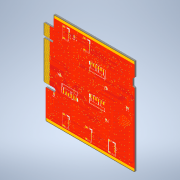
# Autodesk Inventor part: Avionics_PCB
Saved by Autodesk Inventor 2021 (Build 250183000, 183)
## iProperties
Created: 2018-01-15
Part Number: Avionics_PCB
Material: Epoxy Resin
Document SubType Name: Modeling
Designer: Bradley
Density: 1.14 g/cm^3
Appearance: Smooth - Medium Gray
Mass: 15.4834 g
Surface Area: 175.95 cm^2
Volume: 13.582 cm^3
Author: Bradley
Revision Number: 3.1
Autodesk Inventor part; units mm, degrees
ref_plane "XZ Plane" through (0, 0, 0) normal (0, 1, 0) x (-1, 0, 0)
ref_plane "XY Plane" through (0, 0, 0) normal (0, 0, 1) x (1, 0, 0)
sketch "Sketch1" plane through (0, 0, 0) normal (0, 0, 1) x (1, 0, 0)
  line L0 (0, 36.15) -> (10, 36.15)
  line L1 (10, 36.15) -> (10, 47.9)
  line L2 (10, 47.9) -> (90.4, 47.9)
  line L3 (90.4, 47.9) -> (90.4, -47.9)
  line L4 (90.4, -47.9) -> (2, -47.9)
  line L5 (10, -15.15) -> (0, -15.15)
  line L6 (-5.5, 48) -> (90.5, 48) construction
  line L7 (90.5, 48) -> (90.5, -48) construction
  line L8 (90.5, -48) -> (-5.5, -48) construction
  line L9 (-5.5, -48) -> (-5.5, 48) construction
  line L10 (-5.4, 47.9) -> (-3.4, 47.9) construction
  line L11 (-3.4, 47.9) -> (-3.4, -47.9) construction
  line L12 (-3.4, -47.9) -> (-5.4, -47.9) construction
  line L13 (-5.4, -47.9) -> (-5.4, 47.9) construction
  line L14 (-3.4, 38.5) -> (7.85, 38.5) construction
  line L15 (7.85, 38.5) -> (7.85, -17.5) construction
  line L16 (7.85, -17.5) -> (-3.4, -17.5) construction
  line L17 (-3.4, -17.5) -> (-3.4, 38.5) construction
  line L18 (2, -47.9) -> (2, -18.65)
  line L19 (2, -18.65) -> (10, -18.65)
  arc A0 (10, -18.65) -> (10, -15.15) centre (10, -16.9) ccw
  line L20 (0, 24) -> (90.5, 24) construction
  circle A1 centre (-2.5, 47.1) radius 0.9 construction
  circle A2 centre (-0.7, 47.1) radius 0.9 construction
  circle A3 centre (1.1, 47.1) radius 0.9 construction
  circle A4 centre (2.9, 47.1) radius 0.9 construction
  circle A5 centre (4.7, 47.1) radius 0.9 construction
  circle A6 centre (6.5, 47.1) radius 0.9 construction
  circle A7 centre (8.3, 47.1) radius 0.9 construction
  circle A8 centre (-2.5, 45.3) radius 0.9 construction
  circle A9 centre (-0.7, 45.3) radius 0.9 construction
  circle A10 centre (1.1, 45.3) radius 0.9 construction
  circle A11 centre (2.9, 45.3) radius 0.9 construction
  circle A12 centre (4.7, 45.3) radius 0.9 construction
  circle A13 centre (6.5, 45.3) radius 0.9 construction
  circle A14 centre (8.3, 45.3) radius 0.9 construction
  circle A15 centre (-2.5, 43.5) radius 0.9 construction
  circle A16 centre (-0.7, 43.5) radius 0.9 construction
  circle A17 centre (1.1, 43.5) radius 0.9 construction
  circle A18 centre (2.9, 43.5) radius 0.9 construction
  circle A19 centre (4.7, 43.5) radius 0.9 construction
  circle A20 centre (6.5, 43.5) radius 0.9 construction
  circle A21 centre (8.3, 43.5) radius 0.9 construction
  circle A22 centre (-2.5, 41.7) radius 0.9 construction
  circle A23 centre (-0.7, 41.7) radius 0.9 construction
  circle A24 centre (1.1, 41.7) radius 0.9 construction
  circle A25 centre (2.9, 41.7) radius 0.9 construction
  circle A26 centre (4.7, 41.7) radius 0.9 construction
  circle A27 centre (6.5, 41.7) radius 0.9 construction
  circle A28 centre (8.3, 41.7) radius 0.9 construction
  circle A29 centre (-2.5, 39.9) radius 0.9 construction
  circle A30 centre (-0.7, 39.9) radius 0.9 construction
  circle A31 centre (1.1, 39.9) radius 0.9 construction
  circle A32 centre (2.9, 39.9) radius 0.9 construction
  circle A33 centre (4.7, 39.9) radius 0.9 construction
  circle A34 centre (6.5, 39.9) radius 0.9 construction
  circle A35 centre (8.3, 39.9) radius 0.9 construction
  line L21 (0, 36.15) -> (0, 24.95)
  line L22 (0, 24.95) -> (8.4, 24.95)
  arc A36 (8.4, 23.05) -> (8.4, 24.95) centre (8.4, 24) ccw
  line L23 (8.4, 23.05) -> (0, 23.05)
  line L24 (0, 23.05) -> (0, -15.15)
  point P0 (0, 0)
  point P1 (-5.5, 0)
  point P2 (90.4, 0)
  point P3 (90.5, 0)
  dimension "d0" = 51.3
  dimension "d1" = 95.8
  dimension "d3" = 10
  dimension "d20" = 96
  dimension "d21" = 96
  dimension "d22" = 0.1
  dimension "d23" = 0.1
  dimension "d24" = 2
  dimension "d25" = 0.1
  dimension "d28" = 11.25
  dimension "d29" = 56
  dimension "d31" = 9.5
  dimension "d32" = 30.5
  dimension "d34" = 3.5
  dimension "d35" = 12.15
  dimension "d36" = 39.15
  dimension "d37" = 14.5
  dimension "d38" = 1.15
  dimension "d39" = 1.8
  dimension "d42" = 1.8
  dimension "d45" = 1.8
  dimension "d48" = 2
  dimension "d49" = 3.4
  dimension "d50" = 1.9
  dimension "d51" = 8.4
  dimension "d52" = 24
  constraints: 50 end point, 37 centre point, 11 perpendicular, 7 parallel, 6 point on line, 6 tangent, 5 horizontal, 4 point on circle, 3 midpoint, 3 vertical, 2 collinear, 2 horizontal alignment, 68 other
  measures "d0" distance of L5.end L0.start
  measures "d1" distance of L2.end L3.end
  measures "d3" distance of L0.start L0.end
  measures "d20" distance of L6.start L6.end
  measures "d21" distance of L8.end L6.start
  measures "d22" distance between parallel lines of L2 L6
  measures "d23" distance between parallel lines of L7 L3
  measures "d24" distance between parallel lines of L13 L11
  measures "d25" distance between parallel lines of L13 L9
  measures "d28" distance of L15.end L16.end
  measures "d29" distance of L14.end L15.end
  measures "d31" distance between parallel lines of L14 L6
  measures "d32" distance between parallel lines of L8 L16
  measures "d34" distance between parallel lines of L5 L19
  measures "d35" distance between parallel lines of L20 L0
  measures "d36" distance between parallel lines of L5 L20
  measures "d37" distance between parallel lines of L20 L14
  measures "d38" distance between parallel lines of L19 L16
  measures "d39" diameter of A1
  measures "d42" distance of A1.centre A2.centre
  measures "d45" distance of A1.centre A8.centre
  measures "d48" distance between parallel lines of L18 L24
  measures "d49" distance between parallel lines of L24 L11
  measures "d50" distance between parallel lines of L23 L22
  measures "d51" distance of L21.end L22.end
  measures "d52" distance from line of point (0, 0) L20
extrude "Extrusion1" add sketch "Sketch1" along normal mid plane 1.6
chamfer "Chamfer1" distance 0.5 angle 45 4 edges at (0, 36.15, 0) (0, 24.95, 0) (0, 23.05, 0) (0, -15.15, 0)
fillet "Fillet1" radius 0.5 6 edges at (10, 36.15, 0) (10, 47.9, 0) (90.4, 47.9, 0) (90.4, -47.9, 0) (2, -47.9, 0) (2, -18.65, 0)
sketch "Sketch16" plane through (0, 0, 0.8) normal (0, 0, 1) x (1, 0, 0)
  arc A0 (2.5, -18.65) -> (2, -19.15) centre (2.5, -19.15) ccw projected
  line L0 (2, -19.15) -> (2, -47.4) projected
  arc A1 (2, -47.4) -> (2.5, -47.9) centre (2.5, -47.4) ccw projected
  line L1 (2.5, -47.9) -> (89.9, -47.9) projected
  arc A2 (89.9, -47.9) -> (90.4, -47.4) centre (89.9, -47.4) ccw projected
  line L2 (90.4, -47.4) -> (90.4, 47.4) projected
  arc A3 (90.4, 47.4) -> (89.9, 47.9) centre (89.9, 47.4) ccw projected
  line L3 (89.9, 47.9) -> (10.5, 47.9) projected
  arc A4 (10.5, 47.9) -> (10, 47.4) centre (10.5, 47.4) ccw projected
  line L4 (10, 47.4) -> (10, 36.65) projected
  arc A5 (9.5, 36.15) -> (10, 36.65) centre (9.5, 36.65) ccw projected
  line L5 (9.5, 36.15) -> (0.5, 36.15) projected
  line L6 (0, 35.65) -> (0.5, 36.15) projected
  line L7 (0, 35.65) -> (0, 25.45) projected
  line L8 (0.5, 24.95) -> (0, 25.45) projected
  line L9 (0.5, 24.95) -> (8.4, 24.95) projected
  arc A6 (8.4, 23.05) -> (8.4, 24.95) centre (8.4, 24) ccw projected
  line L10 (8.4, 23.05) -> (0.5, 23.05) projected
  line L11 (0, 22.55) -> (0.5, 23.05) projected
  line L12 (0, 22.55) -> (0, -14.65) projected
  line L13 (0.5, -15.15) -> (0, -14.65) projected
  line L14 (0.5, -15.15) -> (10, -15.15) projected
  arc A7 (10, -18.65) -> (10, -15.15) centre (10, -16.9) ccw projected
  line L15 (10, -18.65) -> (2.5, -18.65) projected
  line L16 (90.4, -47.4) -> (90.4, 47.4) projected
  arc A8 (89.4, 33) -> (90.4, 34) centre (89.4, 34) ccw
  arc A9 (89.4, 33) -> (88.4, 32) centre (89.4, 32) ccw
  arc A10 (88.4, 26) -> (89.4, 25) centre (89.4, 26) ccw
  arc A11 (90.4, 24) -> (89.4, 25) centre (89.4, 24) ccw
  line L17 (88.4, 32) -> (88.4, 26)
  line L18 (88.4, 29) -> (90.4, 29) construction
  point P0 (0, 0)
  dimension "d145" = 1
  dimension "d146" = 29
  dimension "d147" = 8
  dimension "d148" = 34
  constraints: 8 point on circle, 6 tangent, 4 centre point, 4 end point, 3 equal radius, 3 point on line, 1 midpoint, 1 perpendicular, 1 vertical, 1 vertical alignment
  measures "d145" radius of A11
  measures "d146" distance from line of L18 point (0, 0)
  measures "d147" distance of A10.end A8.start
  measures "d148" vertical distance of point (0, 0) A8.end
extrude "Extrusion6" cut sketch "Sketch16" against normal through all contours A11 A10 L17 A9 A8 L2
ref_plane "Work Plane1" through (4, 0, 0) normal (1, 0, 0) x (0, 1, 0)
sketch "Sketch17" plane through (4, 0, 0) normal (1, 0, 0) x (0, 1, 0)
  line L0 (-19.15, -0.8) -> (-19.15, 0.8) projected
  line L1 (-47.4, -0.8) -> (-19.15, -0.8) projected
  line L2 (-47.4, 0.8) -> (-47.4, -0.8) projected
  line L3 (-19.15, 0.8) -> (-47.4, 0.8) projected
  point P0 (0, 0)
  point P1 (-42, 1.8)
  point P2 (-41, 1.8)
  point P3 (-40, 1.8)
  point P4 (-39, 1.8)
  point P5 (-42, 2.8)
  point P6 (-41, 2.8)
  point P7 (-40, 2.8)
  point P8 (-39, 2.8)
  point P9 (-42, 3.8)
  point P10 (-41, 3.8)
  point P11 (-40, 3.8)
  point P12 (-39, 3.8)
  point P13 (-42, 4.8)
  point P14 (-41, 4.8)
  point P15 (-40, 4.8)
  point P16 (-39, 4.8)
  dimension "d154" = 1
  dimension "d157" = 1
  dimension "d160" = 42
  dimension "d161" = 1
  constraints: 1 horizontal, 1 vertical, 15 other
  measures "d154" distance of point (-42, 1.8) point (-41, 1.8)
  measures "d157" distance of point (-42, 1.8) point (-42, 2.8)
  measures "d160" horizontal distance of point (-42, 1.8) point (0, 0)
  measures "d161" distance from line of L3 point (-42, 1.8)
sketch "Sketch18" plane through (0, 0, 0) normal (0, 0, 1) x (1, 0, 0)
  arc A0 (90.4, 24) -> (89.4, 25) centre (89.4, 24) ccw projected
  arc A1 (88.4, 26) -> (89.4, 25) centre (89.4, 26) ccw projected
  line L0 (88.4, 26) -> (88.4, 32) projected
  arc A2 (89.4, 33) -> (88.4, 32) centre (89.4, 32) ccw projected
  arc A3 (89.4, 33) -> (90.4, 34) centre (89.4, 34) ccw projected
  line L1 (90.4, 34) -> (90.4, 47.4) projected
  arc A4 (90.4, 47.4) -> (89.9, 47.9) centre (89.9, 47.4) ccw projected
  line L2 (89.9, 47.9) -> (10.5, 47.9) projected
  arc A5 (10.5, 47.9) -> (10, 47.4) centre (10.5, 47.4) ccw projected
  line L3 (10, 47.4) -> (10, 36.65) projected
  arc A6 (9.5, 36.15) -> (10, 36.65) centre (9.5, 36.65) ccw projected
  line L4 (9.5, 36.15) -> (0.5, 36.15) projected
  line L5 (0, 35.65) -> (0.5, 36.15) projected
  line L6 (0, 35.65) -> (0, 25.45) projected
  line L7 (0.5, 24.95) -> (0, 25.45) projected
  line L8 (0.5, 24.95) -> (8.4, 24.95) projected
  arc A7 (8.4, 23.05) -> (8.4, 24.95) centre (8.4, 24) ccw projected
  line L9 (8.4, 23.05) -> (0.5, 23.05) projected
  line L10 (0, 22.55) -> (0.5, 23.05) projected
  line L11 (0, 22.55) -> (0, -14.65) projected
  line L12 (0.5, -15.15) -> (0, -14.65) projected
  line L13 (0.5, -15.15) -> (10, -15.15) projected
  arc A8 (10, -18.65) -> (10, -15.15) centre (10, -16.9) ccw projected
  line L14 (10, -18.65) -> (2.5, -18.65) projected
  arc A9 (2.5, -18.65) -> (2, -19.15) centre (2.5, -19.15) ccw projected
  line L15 (2, -19.15) -> (2, -47.4) projected
  arc A10 (2, -47.4) -> (2.5, -47.9) centre (2.5, -47.4) ccw projected
  line L16 (2.5, -47.9) -> (89.9, -47.9) projected
  arc A11 (89.9, -47.9) -> (90.4, -47.4) centre (89.9, -47.4) ccw projected
  line L17 (90.4, -47.4) -> (90.4, 24) projected
  point P0 (0, 0)
  point P1 (1.5, -44.9)
  point P2 (0.5, -44.9)
  point P3 (1.5, -43.9)
  point P4 (0.5, -43.9)
  point P5 (1.5, -42.9)
  point P6 (0.5, -42.9)
  point P7 (1.5, -41.9)
  point P8 (0.5, -41.9)
  point P9 (1.5, -40.9)
  point P10 (0.5, -40.9)
  point P11 (1.5, -39.9)
  point P12 (0.5, -39.9)
  point P13 (1.5, -38.9)
  point P14 (0.5, -38.9)
  point P15 (1.5, -37.9)
  point P16 (0.5, -37.9)
  point P17 (1.5, -36.9)
  point P18 (0.5, -36.9)
  point P19 (1.5, -35.9)
  point P20 (0.5, -35.9)
  point P21 (1.5, -34.9)
  point P22 (0.5, -34.9)
  point P23 (1.5, -33.9)
  point P24 (0.5, -33.9)
  point P25 (1.5, -32.9)
  point P26 (0.5, -32.9)
  point P27 (1.5, -31.9)
  point P28 (0.5, -31.9)
  point P29 (1.5, -30.9)
  point P30 (0.5, -30.9)
  point P31 (1.5, -29.9)
  point P32 (0.5, -29.9)
  point P33 (1.5, -28.9)
  point P34 (0.5, -28.9)
  point P35 (1.5, -27.9)
  point P36 (0.5, -27.9)
  point P37 (1.5, -26.9)
  point P38 (0.5, -26.9)
  point P39 (1.5, -25.9)
  point P40 (0.5, -25.9)
  point P41 (1.5, -24.9)
  point P42 (0.5, -24.9)
  point P43 (1.5, -23.9)
  point P44 (0.5, -23.9)
  point P45 (1.5, -22.9)
  point P46 (0.5, -22.9)
  point P47 (1.5, -21.9)
  point P48 (0.5, -21.9)
  point P49 (1.5, -20.9)
  point P50 (0.5, -20.9)
  point P51 (9.5, 37.9)
  point P52 (9.5, 38.9)
  point P53 (9.5, 39.9)
  point P54 (9.5, 40.9)
  point P55 (9.5, 41.9)
  point P56 (9.5, 42.9)
  point P57 (9.5, 43.9)
  point P58 (8.5, 37.9)
  point P59 (8.5, 38.9)
  point P60 (8.5, 39.9)
  point P61 (8.5, 40.9)
  point P62 (8.5, 41.9)
  point P63 (8.5, 42.9)
  point P64 (8.5, 43.9)
  point P65 (7.5, 37.9)
  point P66 (7.5, 38.9)
  point P67 (7.5, 39.9)
  point P68 (7.5, 40.9)
  point P69 (7.5, 41.9)
  point P70 (7.5, 42.9)
  point P71 (7.5, 43.9)
  point P72 (6.5, 37.9)
  point P73 (6.5, 38.9)
  point P74 (6.5, 39.9)
  point P75 (6.5, 40.9)
  point P76 (6.5, 41.9)
  point P77 (6.5, 42.9)
  point P78 (6.5, 43.9)
  dimension "d164" = 1
  dimension "d167" = 1
  dimension "d170" = 0.5
  dimension "d171" = 3
  dimension "d172" = 0.5
  dimension "d173" = 10
  dimension "d176" = 1
  dimension "d179" = 1
  constraints: 2 horizontal, 2 vertical, 76 other
  measures "d164" distance of point (1.5, -44.9) point (0.5, -44.9)
  measures "d167" distance of point (1.5, -44.9) point (1.5, -43.9)
  measures "d170" distance from line of L15 point (1.5, -44.9)
  measures "d171" distance from line of L16 point (1.5, -44.9)
  measures "d172" distance from line of point (9.5, 37.9) L3
  measures "d173" distance from line of point (9.5, 37.9) L2
  measures "d176" distance of point (9.5, 37.9) point (9.5, 38.9)
  measures "d179" distance of point (9.5, 37.9) point (8.5, 37.9)
sketch "Sketch19" plane through (0, 0, 0.8) normal (0, 0, 1) x (1, 0, 0)
  line L0 (0, 22.55) -> (0, -14.65) projected
  line L1 (90.4, -47.4) -> (90.4, 24) projected
  line L2 (0, 47.8949) -> (90.4, 47.8949) construction
  line L3 (90.4, 47.8949) -> (90.4, -47.8949) construction
  line L4 (90.4, -47.8949) -> (0, -47.8949) construction
  line L5 (0, -47.8949) -> (0, 47.8949) construction
  point P0 (0, 0)
  constraints: 2 collinear, 1 midpoint, 2 other
decal "Decal3"
sketch "Sketch20" plane through (0, 0, -0.8) normal (0, 0, -1) x (-1, 0, 0)
  line L0 (0, -14.65) -> (0, 22.55) projected
  line L1 (-90.4, 24) -> (-90.4, -47.4) projected
  line L2 (-90.4, 47.8949) -> (0, 47.8949) construction
  line L3 (0, 47.8949) -> (0, -47.8949) construction
  line L4 (0, -47.8949) -> (-90.4, -47.8949) construction
  line L5 (-90.4, -47.8949) -> (-90.4, 47.8949) construction
  point P0 (0, 0)
  constraints: 2 collinear, 1 midpoint, 2 other
decal "Decal4"
sketch "Sketch22" plane through (0, 0, 0.8) normal (0, 0, 1) x (1, 0, 0)
  point P0 (0, 0)
  point P1 (6, 34.5)
  point P2 (6, 32.5)
  point P3 (6, 31.5)
  point P4 (6, 29.5)
  point P5 (6, 28.5)
  point P6 (6, 27.5)
  point P7 (6, 26.5)
  point P8 (6, 25.6)
  point P9 (6, 22.425)
  point P10 (6, 21.5)
  point P11 (6, 20.5)
  point P12 (6, 19.5)
  point P13 (6, 18.5)
  point P14 (6, 17.5)
  point P15 (6, 16.6)
  point P16 (6, 14.5)
  point P17 (6, 13.5)
  point P18 (6, 12.5)
  point P19 (6, 11.5)
  point P20 (87.9, 18.2)
  point P21 (82.2, 16.791)
  point P22 (87.6, 15.5)
  point P23 (25.3, 13.6)
  point P24 (71.8, 15.6)
  point P25 (50.2, 46.1)
  point P26 (46.2, -44.52)
  point P27 (77.9, 4.8)
  point P28 (87.2, -4.3)
  point P29 (49.9, -17.3)
  point P30 (17.6, -12.9)
  point P31 (66.5, -3)
  point P32 (65.93, -8.32)
  point P33 (48.1, 26.5)
  point P34 (66.35, 24.9)
  point P35 (26.962, -21.548)
  point P36 (32.2, -20.55)
  point P37 (65.8, 17.9)
  point P38 (66, 21.9)
  point P39 (15.4, 26.5)
  point P40 (25.9, 16.7)
  point P41 (29.235, 13.76)
  point P42 (33.1, 26.6)
  point P43 (34.7, 23.7)
  point P44 (31.5, 11.8)
  point P45 (20.9, 21.9)
  point P46 (17.7, 22.8)
  point P47 (38.325, 22.345)
  point P48 (10.995, 12.485)
  point P49 (10.995, 11.67)
  point P50 (10.3, 11.7)
  point P51 (24.31, 9)
  point P52 (23.835, 2.255)
  point P53 (33.305, -1.33)
  point P54 (35.5, -3.4)
  point P55 (29.2, -37.9)
  point P56 (46.1, -37.9)
  point P57 (63, -38.5)
  point P58 (79.9, -39.3)
  point P59 (74.3, -38.9)
  point P60 (8.61, -29.3)
  point P61 (23.5, -38.9)
  point P62 (28.3, -31)
  point P63 (39.9, -39)
  point P64 (85.5, -0.8)
  point P65 (57.89, -10.4)
  point P66 (55.74, -17.51)
  point P67 (58.4, -17.7)
  point P68 (64.9, 33.2)
  point P69 (58.25, 10.5)
  point P70 (56.85, 10.5)
  point P71 (77.1, -30.9)
  point P72 (23.425, 25.595)
  point P73 (18.9, 31.2)
  point P74 (35.465, 18.9)
  point P75 (34.135, 15.025)
  point P76 (30.15, 22.355)
  point P77 (57.35, -36.505)
  point P78 (62.1, -30.9)
  point P79 (12.855, -36.35)
  point P80 (45.2, -30.8)
  point P81 (21.925, -18.495)
  point P82 (23.935, -18.495)
  point P83 (26.315, -12.9)
  point P84 (55.3, -0.89)
  point P85 (52.8, -4.31)
  point P86 (45.6, -7.01)
  point P87 (53.275, -18.425)
  point P88 (48.555, 6.31)
  point P89 (51.785, 10.414)
  point P90 (49.681, 11.119)
  point P91 (58.92, 27.11)
  point P92 (56.4, 27.2)
  point P93 (51.67, 28.16)
  point P94 (28.745, -0.49)
  point P95 (45.439, 20.63)
  point P96 (50.617, 22.73)
  point P97 (42.571, 27.565)
  point P98 (39.712, 25.565)
  point P99 (30.035, -16.35)
  point P100 (33.621, -12.379)
  point P101 (15.835, 9)
  point P102 (18.4, -2)
  point P103 (18.4, -5)
  point P104 (24.045, -15.705)
  point P105 (48.7, 31.647)
  point P106 (52.39, 30.62)
  point P107 (70.895, 33.296)
  point P108 (81.9, 40.1)
  point P109 (37.4, 32.3)
  point P110 (24.77, 27.9)
  point P111 (80, -43)
  point P112 (63, -43)
  point P113 (40, -43)
  point P114 (8.5, -42.3)
  point P115 (15, -43)
  point P116 (18, -43)
  point P117 (85, -35)
  point P118 (85, -30)
  point P119 (85, -25)
  point P120 (85, -20)
  point P121 (85, -15)
  point P122 (85, -10)
  point P123 (80, -35)
  point P124 (80, -30)
  point P125 (80, -25)
  point P126 (80, -20)
  point P127 (80, -15)
  point P128 (73.6, -10)
  point P129 (70, -10)
  point P130 (70, -15)
  point P131 (70, -20)
  point P132 (75, -20)
  point P133 (75, -15)
  point P134 (65, -15)
  point P135 (65, -20)
  point P136 (60, -20)
  point P137 (60, -15)
  point P138 (70, -25)
  point P139 (70, -30)
  point P140 (65, -30)
  point P141 (60, -30)
  point P142 (55, -30)
  point P143 (50, -30)
  point P144 (40, -30)
  point P145 (65, -25)
  point P146 (60, -25)
  point P147 (60, -35)
  point P148 (50, -40)
  point P149 (55, -40.1)
  point P150 (35, -30)
  point P151 (35, -25)
  point P152 (25, -30)
  point P153 (30, -30)
  point P154 (30, -40)
  point P155 (21, -40)
  point P156 (20, -30)
  point P157 (15, -30)
  point P158 (15, -34)
  point P159 (5, -30)
  point P160 (5, -25)
  point P161 (5, -20)
  point P162 (15, -25)
  point P163 (20, -20)
  point P164 (25, -25)
  point P165 (30, -25)
  point P166 (30, -20)
  point P167 (35, -20)
  point P168 (45, -20)
  point P169 (40, -20)
  point P170 (40, -15)
  point P171 (45.1, -10)
  point P172 (50, -10)
  point P173 (55, -10)
  point P174 (30, 5)
  point P175 (35, 5)
  point P176 (40, 5)
  point P177 (45, 5)
  point P178 (50.2, 5)
  point P179 (55, 5)
  point P180 (60, 5)
  point P181 (65, 5)
  point P182 (65, 0)
  point P183 (50, 0)
  point P184 (70, 0)
  point P185 (70, -5)
  point P186 (65, 10)
  point P187 (85, 5)
  point P188 (85, 10)
  point P189 (65, 14)
  point P190 (40, 15)
  point P191 (44.7, 15)
  point P192 (35, 15)
  point P193 (40, 10)
  point P194 (35, 10)
  point P195 (30, 10)
  point P196 (25, 10)
  point P197 (10, 15)
  point P198 (15, 15)
  point P199 (15, 20)
  constraints: 744 other
hole "Hole10" at (6, 34.5, 0.8) at (6, 32.5, 0.8) at (6, 31.5, 0.8) at (6, 29.5, 0.8) at (6, 28.5, 0.8) at (6, 27.5, 0.8) at (6, 26.5, 0.8) at (6, 25.6, 0.8) at (6, 22.425, 0.8) at (6, 21.5, 0.8) at (6, 20.5, 0.8) at (6, 19.5, 0.8) at (6, 18.5, 0.8) at (6, 17.5, 0.8) at (6, 16.6, 0.8) at (6, 14.5, 0.8) at (6, 13.5, 0.8) at (6, 12.5, 0.8) at (6, 11.5, 0.8) at (87.9, 18.2, 0.8) at (82.2, 16.791, 0.8) at (87.6, 15.5, 0.8) at (25.3, 13.6, 0.8) at (71.8, 15.6, 0.8) at (50.2, 46.1, 0.8) at (46.2, -44.52, 0.8) at (77.9, 4.8, 0.8) at (87.2, -4.3, 0.8) at (49.9, -17.3, 0.8) at (17.6, -12.9, 0.8) at (66.5, -3, 0.8) at (65.93, -8.32, 0.8) at (48.1, 26.5, 0.8) at (66.35, 24.9, 0.8) at (26.962, -21.548, 0.8) at (32.2, -20.55, 0.8) at (65.8, 17.9, 0.8) at (66, 21.9, 0.8) at (15.4, 26.5, 0.8) at (25.9, 16.7, 0.8) at (29.235, 13.76, 0.8) at (33.1, 26.6, 0.8) at (34.7, 23.7, 0.8) at (31.5, 11.8, 0.8) at (20.9, 21.9, 0.8) at (17.7, 22.8, 0.8) at (38.325, 22.345, 0.8) at (10.995, 12.485, 0.8) at (10.995, 11.67, 0.8) at (10.3, 11.7, 0.8) direction (0, 0, -1) diameter 0.3 end through all and at (24.31, 9, 0.8) (23.835, 2.255, 0.8) (33.305, -1.33, 0.8) (35.5, -3.4, 0.8) (29.2, -37.9, 0.8) (46.1, -37.9, 0.8) (63, -38.5, 0.8) (79.9, -39.3, 0.8) (74.3, -38.9, 0.8) (8.61, -29.3, 0.8) (23.5, -38.9, 0.8) (28.3, -31, 0.8) (39.9, -39, 0.8) (85.5, -0.8, 0.8) (57.89, -10.4, 0.8) (55.74, -17.51, 0.8) (58.4, -17.7, 0.8) (64.9, 33.2, 0.8) (58.25, 10.5, 0.8) (56.85, 10.5, 0.8) (77.1, -30.9, 0.8) (23.425, 25.595, 0.8) (18.9, 31.2, 0.8) (35.465, 18.9, 0.8) (34.135, 15.025, 0.8) (30.15, 22.355, 0.8) (57.35, -36.505, 0.8) (62.1, -30.9, 0.8) (12.855, -36.35, 0.8) (45.2, -30.8, 0.8) (21.925, -18.495, 0.8) (23.935, -18.495, 0.8) (26.315, -12.9, 0.8) (55.3, -0.89, 0.8) (52.8, -4.31, 0.8) (45.6, -7.01, 0.8) (53.275, -18.425, 0.8) (48.555, 6.31, 0.8) (51.785, 10.414, 0.8) (49.681, 11.119, 0.8) (58.92, 27.11, 0.8) (56.4, 27.2, 0.8) (51.67, 28.16, 0.8) (28.745, -0.49, 0.8) (45.439, 20.63, 0.8) (50.617, 22.73, 0.8) (42.571, 27.565, 0.8) (39.712, 25.565, 0.8) (30.035, -16.35, 0.8) (33.621, -12.379, 0.8) (15.835, 9, 0.8) (18.4, -2, 0.8) (18.4, -5, 0.8) (24.045, -15.705, 0.8) (48.7, 31.647, 0.8) (52.39, 30.62, 0.8) (70.895, 33.296, 0.8) (81.9, 40.1, 0.8) (37.4, 32.3, 0.8) (24.77, 27.9, 0.8) (80, -43, 0.8) (63, -43, 0.8) (40, -43, 0.8) (8.5, -42.3, 0.8) (15, -43, 0.8) (18, -43, 0.8) (85, -35, 0.8) (85, -30, 0.8) (85, -25, 0.8) (85, -20, 0.8) (85, -15, 0.8) (85, -10, 0.8) (80, -35, 0.8) (80, -30, 0.8) (80, -25, 0.8) (80, -20, 0.8) (80, -15, 0.8) (73.6, -10, 0.8) (70, -10, 0.8) (70, -15, 0.8) (70, -20, 0.8) (75, -20, 0.8) (75, -15, 0.8) (65, -15, 0.8) (65, -20, 0.8) (60, -20, 0.8) (60, -15, 0.8) (70, -25, 0.8) (70, -30, 0.8) (65, -30, 0.8) (60, -30, 0.8) (55, -30, 0.8) (50, -30, 0.8) (40, -30, 0.8) (65, -25, 0.8) (60, -25, 0.8) (60, -35, 0.8) (50, -40, 0.8) (55, -40.1, 0.8) (35, -30, 0.8) (35, -25, 0.8) (25, -30, 0.8) (30, -30, 0.8) (30, -40, 0.8) (21, -40, 0.8) (20, -30, 0.8) (15, -30, 0.8) (15, -34, 0.8) (5, -30, 0.8) (5, -25, 0.8) (5, -20, 0.8) (15, -25, 0.8) (20, -20, 0.8) (25, -25, 0.8) (30, -25, 0.8) (30, -20, 0.8) (35, -20, 0.8) (45, -20, 0.8) (40, -20, 0.8) (40, -15, 0.8) (45.1, -10, 0.8) (50, -10, 0.8) (55, -10, 0.8) (30, 5, 0.8) (35, 5, 0.8) (40, 5, 0.8) (45, 5, 0.8) (50.2, 5, 0.8) (55, 5, 0.8) (60, 5, 0.8) (65, 5, 0.8) (65, 0, 0.8) (50, 0, 0.8) (70, 0, 0.8) (70, -5, 0.8) (65, 10, 0.8) (85, 5, 0.8) (85, 10, 0.8) (65, 14, 0.8) (40, 15, 0.8) (44.7, 15, 0.8) (35, 15, 0.8) (40, 10, 0.8) (35, 10, 0.8) (30, 10, 0.8) (25, 10, 0.8) (10, 15, 0.8) (15, 15, 0.8) (15, 20, 0.8) (10, 20, 0.8) (10, 25, 0.8) (10, 30, 0.8) (15, 30, 0.8) (15, 25, 0.8) (10, 35, 0.8) (15, 35, 0.8) (20, 35, 0.8) (25, 20, 0.8) (20, 20, 0.8) (30, 35, 0.8) (35, 35, 0.8) (40, 35, 0.8) (44.9, 30, 0.8) (15, 40, 0.8) (20, 40, 0.8) (40, 39, 0.8) (30, 41, 0.8) (55, 41, 0.8) (65, 40, 0.8) (81, 35, 0.8) (80, 30, 0.8) (70, 26, 0.8) (85, 35, 0.8) (85, 40, 0.8) (80, 40, 0.8) (85, -43, 0.8) (75, -43, 0.8) (70, -43, 0.8) (60, -43, 0.8) (55, -43, 0.8) (50, -43, 0.8) (45, -43, 0.8) (35, -43, 0.8) (30, -43, 0.8) (25, -43, 0.8) (85, -39.8, 0.8) (75, -30, 0.8) (75, -35, 0.8) (74, -5, 0.8) (78, 0, 0.8) (50, -34, 0.8) (45, -26, 0.8) (44.855, -0.265, 0.8) (39.9, 1, 0.8) (35, 1, 0.8) (30, 1, 0.8) (35, -34, 0.8) (40, -34, 0.8) (30, -33, 0.8) (25, -33, 0.8) (20, -35, 0.8) (30, 30, 0.8) (30, 25, 0.8) (45, 10, 0.8) (70, 22, 0.8) (75.8, 26, 0.8) (67, 14, 0.8) (67, 10, 0.8) (85, 26, 0.8) (88, 20, 0.8) (88, 25, 0.8) (61, 41, 0.8) (63, 44, 0.8) (38.5, 38.7, 0.8) (11.7, -31, 0.8) (7.165, -31, 0.8) (9.305, -25.593, 0.8) (13.5, -21.3, 0.8) (20.1, -18.6, 0.8) (22.8, -23.5, 0.8) (39.5, -23.4, 0.8) (86.4, -0.8, 0.8) (88.904, 14.104, 0.8) (83.3, 14.1, 0.8) (77.8, 14.1, 0.8) (79.9, 22.7, 0.8) (74.6, 22.7, 0.8) (85.7, 22.7, 0.8) (77.61, -18.5, 0.8) (72.54, -24.1, 0.8) (56.9, -23.5, 0.8) (35.606, 16.853, 0.8) (35.61, 7.4, 0.8) (45.01, 31.8, 0.8) (56.49, 35.745, 0.8) (42.985, 26.789, 0.8) (55.025, -25.2, 0.8) (60.3, 35.7, 0.8) (55.55, 38.9, 0.8) (61.54, -0.695, 0.8) (68.4, 4.5, 0.8) (72.6, 38.2, 0.8) (74.9, 38.3, 0.8) (71.085, 36.91, 0.8) (73.7, 35.745, 0.8) (73.005, 28.355, 0.8) (20.2, 38.26, 0.8) (26.2, 38.9, 0.8) (57.861, 33.475, 0.8) (60.6, 28.6, 0.8) (79, -11, 0.8) (79, -13, 0.8) (78, -14, 0.8) (80, -12, 0.8) (81, -11, 0.8) (82, -10, 0.8) (81, -9, 0.8) (80, -10, 0.8) (79, -9, 0.8) (78, -10, 0.8) (78, -8, 0.8) (80, -8, 0.8) (82, -8, 0.8) (84, -8.1, 0.8) (83, -9, 0.8) (80, -14, 0.8) (81, -13, 0.8) (82, -12, 0.8) (83, -11, 0.8) (84, -10, 0.8) (85, -9, 0.8) (86, -8, 0.8) (85, -7, 0.8) (84, -6, 0.8) (82, -6, 0.8) (80, -6.2, 0.8) (78, -6, 0.8) (75.3, -7.2, 0.8) (77, -12, 0.8) (79.2, -5, 0.8) (80.8, -5, 0.8) (76, -14, 0.8) (74.4, -12.5, 0.8) (74.4, -10.2, 0.8) (74.4, -8.8, 0.8) (62.13, 18.6, 0.8) (57.867, 20.163, 0.8) (54.945, 26.914, 0.8) (53.15, 29.935, 0.8) (51.379, 25.735, 0.8) (48.219, 24.965, 0.8) (50.13, 23.315, 0.8) (46.225, 20.647, 0.8) (70.763, 21.053, 0.8) (46, 19.867, 0.8) (70.175, 20.515, 0.8) (6, -9.5, 0.8) (30.675, -8.99, 0.8) (41.423, -8.723, 0.8) (6, -8.5, 0.8) (30.13, -8.38, 0.8) (40.8, -8.2, 0.8) (52.74, 3.2, 0.8) (80.845, 3.15, 0.8) (57.8, 23.9, 0.8) (53.433, 21.867, 0.8) (53.87, 3.715, 0.8) (72.4, 3.715, 0.8) (53.6, 2.585, 0.8) (70.118, 2.585, 0.8) (82.355, 11.545, 0.8) (57.39, 6.51, 0.8) (81.755, 12.091, 0.8) (59.755, 12.6, 0.8) (76.285, 11.961, 0.8) (60.7, 8.415, 0.8) (76.885, 11.415, 0.8) (60.085, 7.785, 0.8) (75.7, 11.4, 0.8) (54.78, 9, 0.8) (81.2, 11.5, 0.8) (52.173, 7.773, 0.8) (87.545, 12.355, 0.8) (49.221, 16.93, 0.8) (88.16, 12.825, 0.8) (49.8, 17.5, 0.8) (86.97, 12.855, 0.8) (50.431, 16.39, 0.8) (6, -10.5, 0.8) (34.806, -7.84, 0.8) (40.24, -7.685, 0.8) (30.626, -12.315, 0.8) (53.385, 23.565, 0.8) (41.985, 22.935, 0.8) (24.705, 22.925, 0.8) (67.8, 31.2, 0.8) (53.91, 30.635, 0.8) (53.385, 22.755, 0.8) (41.97, 21.79, 0.8) (24.135, 22.07, 0.8) (68.61, 31.183, 0.8) (57.2, 28.1, 0.8) (18.265, 11.5, 0.8) (21.2, 11.5, 0.8) (68.285, 18.99, 0.8) (84.376, 20.034, 0.8) (86.3, 41.9, 0.8) (57.247, 18.917, 0.8) (35.77, 18, 0.8) (70.6, -33.995, 0.8) (67.8, 18.4, 0.8) (83.8, 19.415, 0.8) (84.9, 41.9, 0.8) (57.75, 18.347, 0.8) (37.17, 17.99, 0.8) (71.36, -34.595, 0.8) (87.2, -2.8, 0.8) (76.5, 4.8, 0.8) (53.48, 26.22, 0.8) (50.363, 25.713, 0.8) (48.9, 8.4, 0.8) (46.7, 9.7, 0.8) (51.8, 7, 0.8) (6, 33.5, 0.8) (73.8, 11.4, 0.8) (79.3, 11.4, 0.8) (84.9, 11.4, 0.8) (69.375, 31.22, 0.8) (66.45, 33.54, 0.8) (66.9, 16.045, 0.8) (67.6, 19.9, 0.8) (55.345, 10.49, 0.8) (48.2, 11.2, 0.8) (45.5, 23.9, 0.8) (33.8, 43.7, 0.8) (65.238, 37.538, 0.8) (82.71, 41.35, 0.8) (54.7, 28.81, 0.8) (57.767, 27.593, 0.8) (42.6, 28.4, 0.8) (41.1, 31.2, 0.8) (33.8, 29.1, 0.8) (34.7, 25.1, 0.8) (27.6, 18.1, 0.8) (29.24, 15.02, 0.8) (21.2, 8.4, 0.8) (21.2, 2.5, 0.8) (18.715, 24.86, 0.8) (15.29, 27.95, 0.8) (24.98, 31.545, 0.8) (49.32, 36.9, 0.8) (49.546, 33.285, 0.8) (53.595, 33.261, 0.8) (57.87, 23.134, 0.8) (60.535, 16.05, 0.8) (49.3, 10, 0.8) (73.1, -36.5, 0.8) (34.37, 22.355, 0.8) (75, -9.6, 0.8) (84, 4.9, 0.8) (47.6, 24.46, 0.8) (6.8, -7.8, 0.8) (37.5, -5.21, 0.8) (56.772, -11.673, 0.8) (37.9, -11.579, 0.8) (39.633, -1.37, 0.8) (37.5, -4.44, 0.8) (7.5, -7.285, 0.8) (57.359, -12.241, 0.8) (38.505, -12.25, 0.8) (39, -1.99, 0.8) (37.835, -2.84, 0.8) (8.245, -6.955, 0.8) (57.99, -12.815, 0.8) (39.1, -12.9, 0.8) (38.37, -1.055, 0.8) (37.5, -1.74, 0.8) (9.005, -6.64, 0.8) (56.965, -13.38, 0.8) (39.7, -13.5, 0.8) (51.3, 27.4, 0.8) (48.4, 29, 0.8) (55.355, 23.565, 0.8) (44.665, -15.201, 0.8) (44.88, -1.075, 0.8) (58.802, 1.402, 0.8) (50.367, 14.228, 0.8) (21.3, 10.2, 0.8) (51.519, 14.23, 0.8) (21.2, 4.3, 0.8) (46.038, 15.307, 0.8) (17.03, 25.849, 0.8) (17.335, 29.5, 0.8) (17.1, 16, 0.8) (45.37, 15.965, 0.8) (22.065, 16.3, 0.8) (36.5, 30.4, 0.8) (41.515, 16.51, 0.8) (46, 16.557, 0.8) (36.44, 25.15, 0.8) (45.065, 17.142, 0.8) (41.97, 17.142, 0.8) (40.8, 25.565, 0.8) (41.1, 30.235, 0.8) (46.027, 17.727, 0.8) (29.4, 20.4, 0.8) (33.28, 20.345, 0.8) (45.19, 19.867, 0.8) (54, 36.9, 0.8) (58.2, 36.905, 0.8) (54.195, 9.6, 0.8) (6, -7.5, 0.8) (67.02, -19.32, 0.8) (52.4, -15.9, 0.8) (34.635, -18.56, 0.8) (27, -5.7, 0.8) (30.6, 31, 0.8) (39.435, 30.3, 0.8) (23.265, 31, 0.8) (52.8, 21.242, 0.8) (32.415, 21.245, 0.8) (55.355, 22.64, 0.8) (50.865, 30.575, 0.8) (63.945, 31.175, 0.8) (51.559, 40.4, 0.8) (25.8, 40.4, 0.8) (52.3, 40.975, 0.8) (43.6, 40.94, 0.8) (32.3, 41.01, 0.8) (53.1, 40.975, 0.8) (77.395, 32.516, 0.8) (77.935, 31.727, 0.8) (75.07, 17.29, 0.8) (77.345, 33.915, 0.8) (77.05, 17.285, 0.8) (86.17, 17.276, 0.8) (62.83, 29.125, 0.8) (83.26, 28.8, 0.8) (64.48, 35.601, 0.8) (62.2, 35.6, 0.8) (63.525, 29.438, 0.8) (77.295, 29.435, 0.8) (64.8, 41.36, 0.8) (69.2, 41.36, 0.8) (64.265, 29.775, 0.8) (85.001, 29.9, 0.8) (6, 15.5, 0.8) (73.8, 18.2, 0.8) (79.4, 18.2, 0.8) (85, 18.2, 0.8) (70.8, 16, 0.8) (47.59, 35.73, 0.8) (78.2, 34.4, 0.8) (47.58, 36.49, 0.8) (76.315, 35.34, 0.8) (49.97, 36.485, 0.8) (84.67, 36.595, 0.8) (74, 23.965, 0.8) (79.2, 23.965, 0.8) (85.01, 23.965, 0.8) (63.4, 27.9, 0.8) (73.7, 19, 0.8) (76.635, 33.375, 0.8) (84.271, -41.286, 0.8) (48.7, 42.3, 0.8) (87.06, 41.9, 0.8) (86.4, 0.7, 0.8) (88.84, 0.7, 0.8) (74.91, 37.4, 0.8) (67.568, 37.468, 0.8) (68.4, 40.1, 0.8) (20.2, 37.5, 0.8) (69.2, 40.1, 0.8) (77.055, 40.155, 0.8) (70.803, 40.64, 0.8) (32.945, 37.475, 0.8) (71.73, 40.71, 0.8) (76.46, 40.71, 0.8) (81.7, 5.1, 0.8) (57.982, -8.218, 0.8) (59.035, -0.835, 0.8) (6.61, -40.85, 0.8) (60.7, -2.3, 0.8) (66.475, -5.4, 0.8) (33.5, -33.9, 0.8) (34.4, -21.7, 0.8) (66.26, -21.175, 0.8) (50.6, -4.6, 0.8) (54.47, -5.81, 0.8) (52.445, -1.07, 0.8) (45.6, -3.99, 0.8) (48.07, -23.525, 0.8) (50.75, -23.53, 0.8) (48.828, -24.638, 0.8) (68.836, -36.36, 0.8) (49.595, -24.631, 0.8) (70.8, -24.7, 0.8) (57.931, -2.285, 0.8) (37.39, -0.955, 0.8) (34.94, -4.002, 0.8) (10.6, 0.9, 0.8) (10.8, -12.4, 0.8) (61.057, -16.243, 0.8) (55.025, -13.68, 0.8) (5.875, -42.34, 0.8) (58.375, -35.185, 0.8) (7.245, -44.155, 0.8) (76.5, -44.1, 0.8) (46.6, -14.065, 0.8) (46.019, -15.73, 0.8) (48.9, -17.4, 0.8) (52.84, -19.89, 0.8) (51, -18.2, 0.8) (54.122, -17.578, 0.8) (56.11, -20.665, 0.8) (36.4, -3.4, 0.8) (36.5, -6.4, 0.8) (50.655, 29.06, 0.8) (53.7, 28.1, 0.8) (6, 30.5, 0.8) (57.548, -11.133, 0.8) (55.944, -13.68, 0.8) (55.2, -38.9, 0.8) (62.2, -39.4, 0.8) (72.1, -39.485, 0.8) (80.7, -40.1, 0.8) (56.165, -16.6, 0.8) (58.59, -4.7, 0.8) (58.09, -1.3, 0.8) (45.6, -2.59, 0.8) (47.1, 26.5, 0.8) (45.567, 0.115, 0.8) (44.065, 2.609, 0.8) (44.065, 24.3, 0.8) (21.344, -14.8, 0.8) (26.319, -15.735, 0.8) (6, 0.5, 0.8) (25.292, -4.908, 0.8) (6, -0.5, 0.8) (24.71, -5.4, 0.8) (18.3, -24.824, 0.8) (19.7, -24.9, 0.8) (22.695, -11.68, 0.8) (36.715, -11.875, 0.8) (17.6, -11.5, 0.8) (50.71, -20.74, 0.8) (53.885, -20.735, 0.8) (33.3, -2.9, 0.8) (33.9, -6.1, 0.8) (49.6, 7.1, 0.8) (46.4, 7.1, 0.8) (6, 35.5, 0.8) (10.1, -39.1, 0.8) (11.026, -34.535, 0.8) (21.502, -38.902, 0.8) (16.7, -20.2, 0.8) (22.23, -20.75, 0.8) (29.2, -39.4, 0.8) (37.705, -38.985, 0.8) (46.1, -39.6, 0.8) (23.745, -13.7, 0.8) (30.795, -14.733, 0.8) (34.403, -13.897, 0.8) (29.535, -1.2, 0.8) (20.3, -4.6, 0.8) (7, 10.5, 0.8) (26.2, 4.9, 0.8) (7, 9.5, 0.8) (25.072, 4.865, 0.8) (7, 8.5, 0.8) (23.172, 4.865, 0.8) (7, 7.5, 0.8) (22.362, 4.865, 0.8) (11.724, -3.976, 0.8) (13.15, -2.15, 0.8) (12, -4.835, 0.8) (13.3, -3.5, 0.8) (30.45, -5.76, 0.8) (29.3, -12.315, 0.8) (29.084, -7.806, 0.8) (28.086, -12.315, 0.8) (29.644, -11.235, 0.8) (34.165, -14.962, 0.8) (6, 4.5, 0.8) (6, 3.5, 0.8) (21.2, 1.7, 0.8) (6, 2.5, 0.8) (15.82, 2.495, 0.8) (15.9, -0.125, 0.8) (26.815, 0.413, 0.8) (15.9, 1.065, 0.8) (17.6, -1.665, 0.8) (14.4, -38.5, 0.8) (7.3, -38.5, 0.8) (9.265, -37.935, 0.8) (12.665, -34.535, 0.8) (7.075, -30.075, 0.8) (7, -25.5, 0.8) (5.33, -41.045, 0.8) (23.795, -34.515, 0.8) (4.1, -40.9, 0.8) (40.9, -34.62, 0.8) (9.121, -39.065, 0.8) (4.57, -35.27, 0.8) (32.8, 39.21, 0.8) (80.235, 24.9, 0.8) (86.035, 24.9, 0.8) (75, 24.9, 0.8) (54.36, 33.223, 0.8) (75, 41.335, 0.8) (73.585, 31.612, 0.8) (61.9, 33.515, 0.8) (38.6, 41.7, 0.8) (59.4, 41.7, 0.8) (61.9, 31.792, 0.8) (57.895, 31.792, 0.8) (56.5, 33.7, 0.8) (11.3, -19.1, 0.8) (6, -1.5, 0.8) (25.79, -5.985, 0.8) (6, -2.5, 0.8) (21.2, -9.61, 0.8) (42.636, -9.564, 0.8) (42.041, -22.371, 0.8) (54.5, -21.9, 0.8) (12.3, -9.63, 0.8) (6, -3.5, 0.8) (21.74, -10.145, 0.8) (41.463, -10.137, 0.8) (41.463, -22.948, 0.8) (55.223, -22.523, 0.8) (12.881, -10.195, 0.8) (6, -4.5, 0.8) (21.2, -10.69, 0.8) (40.89, -10.71, 0.8) (38.085, -21.905, 0.8) (51.665, -21.83, 0.8) (12.3, -10.76, 0.8) (6, 1.5, 0.8) (35.626, -6.674, 0.8) (30.782, -6.682, 0.8) (54.1, -36.5, 0.8) (56.4, -36.5, 0.8) (59.71, 10.5, 0.8) (52.9, -24.066, 0.8) (44.1, -23.513, 0.8) (44.07, -1.085, 0.8) (31.395, 0.095, 0.8) (23.315, -5.953, 0.8) (6.849, -5.135, 0.8) (24.7, -2.1, 0.8) (21.385, -1.201, 0.8) (19.981, -2.619, 0.8)
equation "\"d23\" = d22"
equation "\"d25\" = d22"
equation "\"d42\" = d39"
equation "\"d45\" = d39"
body "Solid1"
